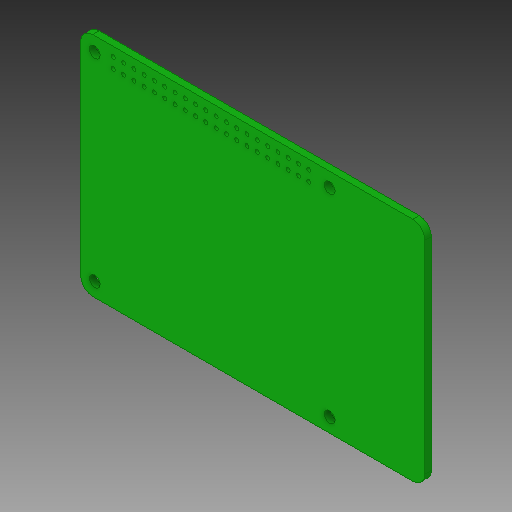
# Autodesk Inventor part: RasPiArm基板
Saved by Autodesk Inventor 2017 (Build 210142000, 142)
## iProperties
Created: 2016-08-20
Part Number: RasPiArm基板
Material: GFRC
Document SubType Name: Modeling
Designer: NN
Density: 1.7 g/cm^3
Appearance: 濃い緑
Mass: 12.7784 g
Surface Area: 100.942 cm^2
Volume: 7.51673 cm^3
Author: NN
Autodesk Inventor part; units mm, degrees
ref_plane "YZ Plane" through (0, 0, 0) normal (1, 0, 0) x (0, 1, 0)
ref_plane "XZ Plane" through (0, 0, 0) normal (0, 1, 0) x (-1, 0, 0)
ref_plane "XY Plane" through (0, 0, 0) normal (0, 0, 1) x (1, 0, 0)
sketch "スケッチ1" plane through (0, 0, 0) normal (0, 0, 1) x (1, 0, 0)
  line L0 (0, 0) -> (85, 0)
  line L1 (85, 0) -> (85, 56)
  line L2 (85, 56) -> (0, 56)
  line L3 (0, 56) -> (0, 0)
  dimension "d0" = 56
  dimension "d1" = 85
  constraints: 8 end point, 2 parallel, 1 horizontal, 1 perpendicular
  measures "d0" distance of L2.end L0.start
  measures "d1" distance of L0.start L0.end
extrude "押し出し1" add sketch "スケッチ1" along normal blind 1.6
fillet "フィレット1" radius 3 4 edges at (85, 56, 0.8) (85, 0, 0.8) (0, 0, 0.8) (0, 56, 0.8)
sketch "スケッチ2" plane through (0, 0, 1.6) normal (0, 0, 1) x (1, 0, 0)
  line L0 (3.5, 52.5) -> (61.5, 52.5)
  line L1 (61.5, 52.5) -> (61.5, 3.5)
  line L2 (61.5, 3.5) -> (3.5, 3.5)
  line L3 (3.5, 3.5) -> (3.5, 52.5)
  line L4 (0, 53) -> (0, 3) projected
  line L5 (0, 28) -> (3.5, 28)
  point P0 (0, 0)
  dimension "d5" = 58
  dimension "d6" = 49
  dimension "d7" = 3.5
  constraints: 10 end point, 2 midpoint, 2 parallel, 2 perpendicular, 1 horizontal
  measures "d5" distance of L1.end L2.end
  measures "d6" distance of L0.end L1.end
  measures "d7" distance between parallel lines of L4 L3
hole "穴1" at (61.5, 52.5, 1.6) at (61.5, 3.5, 1.6) at (3.5, 3.5, 1.6) at (3.5, 52.5, 1.6) direction (0, 0, -1) diameter 2.7 end through all
sketch "スケッチ3" plane through (0, 0, 1.6) normal (0, 0, 1) x (1, 0, 0)
  circle A0 centre (8.07, 53.77) radius 0.5
  line L0 (82, 56) -> (3, 56) projected
  line L1 (0, 53) -> (0, 3) projected
  point P0 (0, 0)
  dimension "d15" = 1
  dimension "d16" = 2.23
  dimension "d17" = 8.07
  constraints: 1 centre point
  measures "d15" diameter of A0
  measures "d16" distance from line of L0 A0.centre
  measures "d17" distance from line of A0.centre L1
hole "穴2" at (8.07, 53.77, 1.6) direction (0, 0, -1) diameter 1 end through all
pattern_linear "矩形状パターン1" count 2 spacing 2.54 along (0, -1, 0) count 20 spacing 2.54 along (1, 0, 0) of "穴2"
